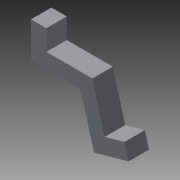
# Autodesk Inventor part: AttachmentPlateHopper_v1
Saved by Autodesk Inventor 2013 (Build 170138000, 138)
## iProperties
Created: 2013-01-16
Part Number: AttachmentPlateHopper_v1
Material: Generic
Document SubType Name: Modeling
Designer: twsass
Density: 1 g/cm^3
Author: twsass
Autodesk Inventor part; units mm, degrees
ref_plane "YZ Plane" through (0, 0, 0) normal (1, 0, 0) x (0, 1, 0)
ref_plane "XZ Plane" through (0, 0, 0) normal (0, 1, 0) x (-1, 0, 0)
ref_plane "XY Plane" through (0, 0, 0) normal (0, 0, 1) x (1, 0, 0)
sketch "Sketch1" plane through (0, 0, 0) normal (0, 0, 1) x (1, 0, 0)
  line L0 (0, 0) -> (0, 9.525)
  line L1 (9.525, 9.525) -> (38.1, 9.525)
  line L2 (38.1, 9.525) -> (45.7363, -18.0107)
  line L3 (38.1, 9.525) -> (76.2, 9.525) construction
  line L4 (48.2818, -27.1893) -> (39.1032, -29.7348)
  line L5 (39.1032, -29.7348) -> (30.857, 0)
  line L6 (30.857, 0) -> (0, 0)
  line L7 (48.2818, -27.1893) -> (60.5199, -23.7954)
  line L8 (60.5199, -23.7954) -> (57.9744, -14.6168)
  line L9 (57.9744, -14.6168) -> (45.7363, -18.0107)
  line L10 (0, 9.525) -> (0, 22.225)
  line L11 (0, 22.225) -> (9.525, 22.225)
  line L12 (9.525, 22.225) -> (9.525, 9.525)
  dimension "d0" = 9.525
  dimension "d1" = 38.1
  dimension "d2" = 38.1
  dimension "d3" = 74.5
  dimension "d4" = 9.525
  dimension "d24" = 12.7
  dimension "d25" = 9.525
  dimension "d26" = 12.7
  dimension "d27" = 9.525
  constraints: 26 end point, 8 perpendicular, 1 horizontal, 1 parallel, 1 point on line, 1 vertical
  measures "d0" distance of L0.start L0.end
  measures "d1" distance of L0.end L1.end
  measures "d2" distance of L1.end L4.start
  measures "d3" angle of L2 L3
  measures "d4" distance of L4.start L4.end
  measures "d24" distance of L4.start L7.end
  measures "d25" distance of L7.end L8.end
  measures "d26" distance of L0.end L10.end
  measures "d27" distance of L10.end L11.end
extrude "Extrusion1" add sketch "Sketch1" along normal blind 12.7
body "Solid1"
